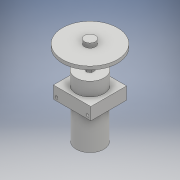
# Autodesk Inventor part: Joinmax
Saved by Autodesk Inventor 2018 (Build 220112000, 112)
## iProperties
Created: 2018-06-13
Part Number: Joinmax
Material: Generic
Document SubType Name: Modeling
Designer: matth
Density: 1 g/cm^3
Appearance: Default
Author: matth
Autodesk Inventor part; units mm, degrees
ref_plane "YZ Plane" through (0, 0, 0) normal (1, 0, 0) x (0, 1, 0)
ref_plane "XZ Plane" through (0, 0, 0) normal (0, 1, 0) x (-1, 0, 0)
ref_plane "XY Plane" through (0, 0, 0) normal (0, 0, 1) x (1, 0, 0)
sketch "Sketch1" plane through (0, 0, 0) normal (0, 0, 1) x (1, 0, 0)
  line L0 (0, 0) -> (17, 0)
  line L1 (17, 0) -> (17, 16.25)
  line L2 (17, 16.25) -> (0, 16.25)
  line L3 (17, 16.25) -> (-17, 16.25)
  line L4 (-17, 16.25) -> (-17, -16.25)
  line L5 (-17, -16.25) -> (17, -16.25)
  line L6 (17, -16.25) -> (17, 16.25)
  dimension "d0" = 17
  dimension "d1" = 16.25
  dimension "d2" = 34
  dimension "d3" = 32.5
  constraints: 14 end point, 3 parallel, 2 horizontal, 2 perpendicular
  measures "d0" distance of L2.end L1.end
  measures "d1" distance of L1.end L0.end
  measures "d2" distance of L5.end L4.end
  measures "d3" distance of L4.end L3.end
extrude "Extrusion1" add sketch "Sketch1" along normal blind 11.25
sketch "Sketch2" plane through (0, 0, 11.25) normal (0, 0, 1) x (1, 0, 0)
  point P0 (0, 0)
sketch "Sketch3" plane through (-17, 16.25, 0) normal (0, 1, 0) x (1, 0, 0)
  line L0 (0, 0) -> (0, -11.25) projected
  line L1 (0, 0) -> (0, -2.9)
  line L2 (0, -2.9) -> (2.9, -2.9)
  line L3 (34, 0) -> (34, -11.25) projected
  line L4 (34, 0) -> (34, -2.9)
  line L5 (34, -2.9) -> (31.1, -2.9)
  circle A0 centre (31.1, -2.9) radius 1.25
  circle A1 centre (2.9, -2.9) radius 1.25
  point P0 (17, 0)
  dimension "d6" = 2.9
  dimension "d7" = 2.9
  dimension "d8" = 2.9
  dimension "d9" = 2.9
  dimension "d10" = 2.5
  dimension "d11" = 2.5
  constraints: 8 end point, 2 centre point, 2 coincident, 2 perpendicular, 2 point on line
  measures "d6" distance of L0.start L1.end
  measures "d7" distance of L1.end L2.end
  measures "d8" distance of L3.start L4.end
  measures "d9" distance of L4.end L5.end
  measures "d10" diameter of A0
  measures "d11" diameter of A1
extrude "Extrusion2" cut sketch "Sketch3" against normal blind 32.5
sketch "Sketch4" plane through (0, 0, 11.25) normal (0, 0, 1) x (1, 0, 0)
  circle A0 centre (0, 0) radius 12.85
  dimension "d14" = 25.7
  constraints: 1 centre point, 1 coincident
  measures "d14" diameter of A0
extrude "Extrusion3" add sketch "Sketch4" along normal blind 12.4
sketch "Sketch5" plane through (0, 0, 23.65) normal (0, 0, 1) x (1, 0, 0)
  circle A0 centre (0, 0) radius 1.5
  line L0 (0, 0) -> (3.5, 0) construction
  line L1 (0, 0) -> (3.5, 0) construction
  line L2 (0, 0) -> (3.5, 0) construction
  line L3 (0, 0) -> (3.5, 0) construction
  line L4 (-3.0311, -1.75) -> (-3.0311, 1.75)
  line L5 (-3.0311, 1.75) -> (0, 3.5)
  line L6 (0, 3.5) -> (3.0311, 1.75)
  line L7 (3.0311, 1.75) -> (3.0311, -1.75)
  line L8 (3.0311, -1.75) -> (0, -3.5)
  line L9 (0, -3.5) -> (-3.0311, -1.75)
  dimension "d17" = 3
  dimension "d18" = 3.5
  dimension "d19" = 3.5
  dimension "d20" = 3.5
  dimension "d22" = 3.5
  dimension "d24" = 3.5
  dimension "d26" = 3.5
  constraints: 20 end point, 4 horizontal, 1 centre point, 1 coincident
  measures "d17" diameter of A0
  measures "d18" distance of L0.start L5.end
  measures "d19" distance of L0.start L8.end
  measures "d20" distance of L0.start L6.end
  measures "d22" distance of L0.start L7.end
  measures "d24" distance of L0.start L4.end
  measures "d26" distance of L0.start L4.start
extrude "Extrusion4" add sketch "Sketch5" along normal blind 11.5
sketch "Sketch6" plane through (0, 0, 0) normal (0, 0, -1) x (-1, 0, 0)
  circle A0 centre (0, 0) radius 12.5
  dimension "d30" = 25
  constraints: 1 centre point, 1 coincident
  measures "d30" diameter of A0
extrude "Extrusion5" add sketch "Sketch6" along normal blind 32.85
sketch "Sketch7" plane through (0, 0, 35.15) normal (0, 0, 1) x (1, 0, 0)
  circle A0 centre (0, 0) radius 1.5 projected
  circle A1 centre (0, 0) radius 5
  dimension "d33" = 10
  constraints: 1 centre point, 1 coincident
  measures "d33" diameter of A1
extrude "Extrusion6" add sketch "Sketch7" along normal blind 6 contours A0 | A1
sketch "Sketch8" plane through (0, 0, 41.15) normal (0, 0, 1) x (1, 0, 0)
  circle A0 centre (0, 0) radius 5 projected
  circle A1 centre (0, 0) radius 25
  dimension "d36" = 50
  constraints: 1 centre point, 1 coincident
  measures "d36" diameter of A1
extrude "Extrusion7" add sketch "Sketch8" along normal blind 3 contours A0 | A1
sketch "Sketch9" plane through (0, 0, 44.15) normal (0, 0, 1) x (1, 0, 0)
  circle A0 centre (0, 0) radius 5
  constraints: 1 centre point, 1 coincident
extrude "Extrusion8" add sketch "Sketch9" along normal blind 4
body "Solid1"
